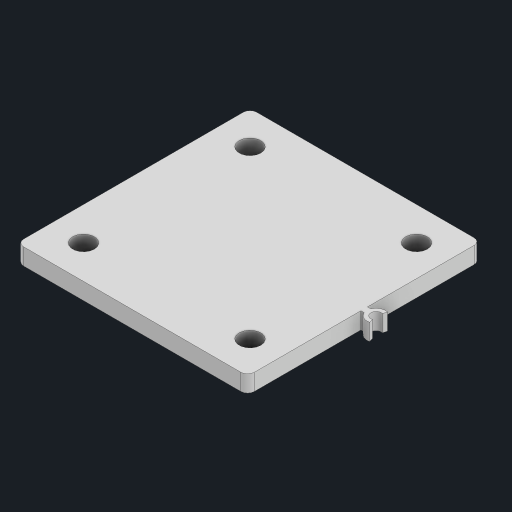
# Autodesk Inventor part: cradle_slider
Saved by Autodesk Inventor 2024 (Build 280153000, 153)
## iProperties
Created: 2024-06-23
Part Number: cradle_slider
Material: Generic
Document SubType Name: Modeling
Designer: mihir
Density: 1 g/cm^3
Appearance: Default
Author: mihir
Autodesk Inventor part; units mm, degrees
ref_plane "YZ Plane" through (0, 0, 0) normal (1, 0, 0) x (0, 1, 0)
ref_plane "XZ Plane" through (0, 0, 0) normal (0, 1, 0) x (-1, 0, 0)
ref_plane "XY Plane" through (0, 0, 0) normal (0, 0, 1) x (1, 0, 0)
sketch "Sketch1" plane through (0, 0, 0) normal (0, 1, 0) x (-1, 0, 0)
  line L0 (-34.6421, 35) -> (34.6421, 35)
  line L1 (34.6421, 35) -> (34.6421, -35)
  line L2 (34.6421, -35) -> (-34.6421, -35)
  line L3 (-34.6421, -35) -> (-34.6421, 35)
  line L4 (-34.6421, 35) -> (34.6421, -35) construction
  line L5 (34.6421, 35) -> (-34.6421, -35) construction
  point P0 (0, 0)
  dimension "d0" = 70
  constraints: 12 end point, 2 midpoint, 2 parallel, 1 horizontal, 1 perpendicular
  measures "d0" distance of L0.end L1.end
extrude "Extrusion1" add sketch "Sketch1" along normal blind 5
fillet "Fillet1" radius 2 4 edges at (-34.6421, 2.5, -35) (-34.6421, 2.5, 35) (34.6421, 2.5, 35) (34.6421, 2.5, -35)
sketch "Sketch2" plane through (0, 0, 0) normal (0, -1, 0) x (1, 0, 0)
  line L0 (36.6421, 1) -> (34.6421, 1)
  line L1 (34.6421, 1) -> (34.6421, -1)
  line L2 (34.6421, -1) -> (36.6421, -1)
  line L3 (36.6421, -1) -> (36.6421, 1)
  line L4 (36.6421, 1) -> (34.6421, -1) construction
  line L5 (34.6421, 1) -> (36.6421, -1) construction
  arc A0 (38.6405, 1.5334) -> (38.6405, -1.5334) centre (38.2296, 0) ccw
  line L6 (34.6421, 33) -> (34.6421, -33) projected
  line L7 (35.6421, 0) -> (34.6421, 0) construction
  arc A1 (38.9511, 2.6925) -> (38.9511, -2.6925) centre (38.2296, 0) ccw
  line L8 (38.9511, 2.6925) -> (38.6405, 1.5334)
  line L9 (38.6405, -1.5334) -> (38.9511, -2.6925)
  point P0 (0, 0)
  point P1 (36.6421, 0)
  point P2 (35.6277, 1)
  point P3 (35.6277, -1)
  dimension "d4" = 150
  dimension "d5" = 1.5875
  dimension "d6" = 2
  dimension "d8" = 150
  dimension "d9" = 1.2
  constraints: 18 end point, 6 midpoint, 5 point on circle, 2 centre point, 2 equal length, 2 parallel, 2 perpendicular, 1 collinear, 1 concentric, 1 horizontal, 1 tangent
  measures "d5" radius of A0
  measures "d6" distance of L0.end L1.end
  measures "d9" radial gap between concentric circles of A1 A0
extrude "Extrusion2" add sketch "Sketch2" against normal up to surface (5 mm away)
sketch "Sketch3" plane through (0, 5, 0) normal (0, 1, 0) x (1, 0, 0)
  circle A0 centre (-24.6421, -25) radius 3.25
  line L0 (-34.6421, 33) -> (-34.6421, -33) projected
  line L1 (-32.6421, -35) -> (32.6421, -35) projected
  circle A1 centre (-24.6421, 25) radius 3.25
  circle A2 centre (25.3579, -25) radius 3.25
  circle A3 centre (25.3579, 25) radius 3.25
  point P0 (0, 0)
  dimension "d12" = 6.5
  dimension "d15" = 50
  dimension "d18" = 50
  dimension "d21" = 10
  dimension "d22" = 10
  constraints: 4 centre point, 1 horizontal, 1 vertical, 6 other
  measures "d12" diameter of A0
  measures "d15" distance of A0.centre A1.centre
  measures "d18" distance of A0.centre A2.centre
  measures "d21" distance from line of L1 A0.centre
  measures "d22" distance from line of L0 A0.centre
extrude "Extrusion3" cut sketch "Sketch3" against normal up to surface (5 mm away)
equation "\"d0\" = cradle_width"
equation "\"d1\" = cradle_slider_thickness"
equation "\"d5\" = 0.5 * tubing_diameter"
equation "\"d10\" = cradle_slider_thickness"
equation "\"d12\" = rod_diameter + rod_free_tolerance"
equation "\"d15\" = rod_dist"
equation "\"d18\" = rod_dist"
equation "\"d21\" = -0.5 * rod_dist + 0.5 * cradle_width"
equation "\"d22\" = -0.5 * rod_dist + 0.5 * cradle_width"
equation "\"cradle_width\" = 70"
equation "\"cradle_slider_thickness\" = 5"
equation "\"tubing_diameter\" = 3.175"
equation "\"rod_diameter\" = 6"
equation "\"rod_free_tolerance\" = 0.5"
equation "\"tube_diameter\" = 15"
equation "\"tube_tip_diameter\" = 5"
equation "\"rod_dist\" = 50"
body "Solid1"
